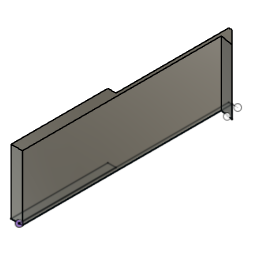
Fermaporte V2 v15 (Autodesk Fusion 360 design; units mm, degrees)
Autodesk Fusion 360 part; units mm, degrees
sketch "Schizzo3" plane through (0, 0, 0) normal (0, 0, 1) x (1, 0, 0)
  line L0 (0, 0) -> (1, 0)
  line L1 (1, 0) -> (1, 65)
  line L2 (1, 65) -> (0, 65)
  line L3 (0, 65) -> (0, 0)
  line L4 (0, 0) -> (-2.5, 0)
  line L5 (-2.5, 0) -> (-2.5, 30)
  line L6 (-2.5, 30) -> (0, 30)
  line L7 (0, 30) -> (0, 0)
  line L8 (1, 65) -> (5, 61)
  line L9 (1, 65) -> (2.8028, 65) construction
  line L10 (5, 61) -> (1, 61.7053)
  line L11 (5, 61) -> (3.5037, 61) construction
  dimension "d7" = 1
  dimension "d8" = 65
  dimension "d9" = 2.5
  dimension "d10" = 30
  dimension "d11" = 45
  dimension "d12" = 190
  dimension "d13" = 4
  constraint horizontal L0
  constraint vertical L1
  constraint horizontal L2
  constraint vertical L3
  constraint coincident L0.start L3.end
  constraint horizontal L4
  constraint vertical L5
  constraint horizontal L6
  constraint vertical L7
  constraint horizontal L9
  constraint horizontal L11
  constraint coincident L1 L10.end
  measures "d7" distance of L0.start L0.end
  measures "d8" distance of L0.start L2.end
  measures "d9" distance of L0.start L4.end
  measures "d10" distance of L0.start L6.end
  measures "d11" angle of L8 L9
  measures "d13" horizontal distance of L1.end L8.end
form "Forma1" [no effect]
extrude "Estrusione2" add sketch "Schizzo3" along normal blind 20
sketch "Schizzo1" plane through (0, 0, 0) normal (0, 0, 1) x (1, 0, 0)
  line L0 (0, 0) -> (1, 0)
  line L1 (1, 0) -> (1, 80)
  line L2 (1, 80) -> (0, 80)
  line L3 (0, 80) -> (0, 0)
  line L4 (0, 63.9506) -> (-8, 71.9506)
  line L5 (0, 63.9506) -> (2.2966, 63.9506) construction
  line L6 (-8, 71.9506) -> (0, 79.9506)
  dimension "d1" = 1
  dimension "d2" = 80
  dimension "d3" = 135
  dimension "d4" = 8
  constraint horizontal L0
  constraint vertical L1
  constraint horizontal L2
  constraint vertical L3
  constraint coincident L0.start L3.end
  constraint horizontal L5
  constraint coincident L3 L4.start
  constraint perpendicular L4 L6
  constraint coincident L3 L6.end
  measures "d1" distance of L0.start L0.end
  measures "d2" distance of L0.start L2.end
  measures "d3" angle of L4 L5
  measures "d4" horizontal distance of L2.end L4.end
extrude "Estrusione1" [suppressed]
equation "d8 = 90 mm - 25 mm"
